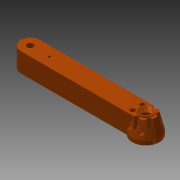
# Autodesk Inventor part: xy ubis mount arm mod
Saved by Autodesk Inventor 2013 (Build 170138000, 138)
## iProperties
Created: 2013-07-23
Part Number: xy ubis mount arm mod
Material: Generic
Document SubType Name: Modeling
Designer: employee
Density: 1 g/cm^3
Mass: 100.24 g
Surface Area: 228.044 cm^2
Volume: 100.24 cm^3
Author: employee
Autodesk Inventor part; units mm, degrees
ref_plane "YZ Plane" through (0, 0, 0) normal (1, 0, 0) x (0, 1, 0)
ref_plane "XZ Plane" through (0, 0, 0) normal (0, 1, 0) x (-1, 0, 0)
ref_plane "XY Plane" through (0, 0, 0) normal (0, 0, 1) x (1, 0, 0)
sketch "Sketch1" plane through (0, 0, 0) normal (0, 0, 1) x (1, 0, 0)
  line L0 (0, 12.5) -> (150, 12.5)
  line L1 (150, -12.5) -> (0, -12.5)
  arc A0 (0, 12.5) -> (0, -12.5) centre (0, 0) ccw
  circle A1 centre (0, 0) radius 4.05
  arc A2 (150, -12.5) -> (150, 12.5) centre (150, 0) ccw
  dimension "d0" = 12.5
  dimension "d3" = 8.1
  dimension "d121" = 150
  constraints: 4 end point, 4 point on circle, 4 tangent, 3 centre point, 2 coincident, 1 horizontal, 1 parallel
  measures "d0" radius of A0
  measures "d3" diameter of A1
  measures "d121" distance of A2.centre point (0, 0)
extrude "Extrusion1" add sketch "Sketch1" along normal blind 25
sketch "Sketch5" plane through (0, 0, 0) normal (0, 0, -1) x (-1, 0, 0)
  line L0 (0, 12.5) -> (-162.5, 12.5)
  line L1 (-162.5, 12.5) -> (-162.5, -12.5)
  line L2 (-162.5, -12.5) -> (0, -12.5)
  circle A0 centre (-150, 0) radius 12.5
  circle A1 centre (-150, 0) radius 8.1
  arc A2 (-162.5, 12.5) -> (-162.5, -12.5) centre (-150, 0) ccw projected
  dimension "d19" = 16.2
  constraints: 6 end point, 3 tangent, 2 centre point, 2 coincident, 1 other
  measures "d19" diameter of A1
extrude "Extrusion5" cut sketch "Sketch5" against normal blind 19 contours A1
sketch "Sketch17" plane through (0, 0, 0) normal (0, 0, -1) x (-1, 0, 0)
  line L0 (0, 12.5) -> (-150, 12.5) projected
  circle A0 centre (0, 0) radius 4.05 projected
  line L1 (0, 0) -> (-25, 0)
  circle A1 centre (-25, 0) radius 1.5
  point P0 (-154.6624, 12.5)
  point P1 (-154.5, 12.5)
  dimension "d85" = 25
  dimension "d86" = 3
  constraints: 2 end point, 1 centre point, 1 coincident, 1 parallel
  measures "d85" distance of L1.start L1.end
  measures "d86" diameter of A1
extrude "Extrusion16" cut sketch "Sketch17" against normal through all contours A1
sketch "Sketch26" plane through (0, 0, 25) normal (0, 0, 1) x (1, 0, 0)
  arc A0 (150, -12.5) -> (150, 12.5) centre (150, 0) ccw projected
  circle A1 centre (150, 0) radius 9
  dimension "d122" = 18
  constraints: 1 centre point, 1 coincident
  measures "d122" diameter of A1
extrude "Extrusion24" add sketch "Sketch26" along normal blind 1.5
sketch "Sketch27" plane through (0, 0, 0) normal (0, 1, 0) x (-1, 0, 0)
  line L0 (-4.05, 25) -> (-4.05, 0) projected
  line L1 (-4.05, 0) -> (-23.5, 0) projected
  line L2 (-23.5, 0) -> (-23.5, 25) projected
  line L3 (-23.5, 25) -> (-4.05, 25) projected
  line L4 (-162.5, 0) -> (-162.5, 25) projected
  line L5 (-162.5, 25) -> (-159, 25) projected
  line L6 (-159, 25) -> (-159, 26.5) projected
  line L7 (-159, 26.5) -> (-141, 26.5) projected
  line L8 (-141, 26.5) -> (-141, 25) projected
  line L9 (-141, 25) -> (-26.5, 25) projected
  line L10 (-26.5, 25) -> (-26.5, 0) projected
  line L11 (-26.5, 0) -> (-141.9, 0) projected
  line L12 (-141.9, 0) -> (-141.9, 19) projected
  line L13 (-141.9, 19) -> (-158.1, 19) projected
  line L14 (-158.1, 19) -> (-158.1, 0) projected
  line L15 (-158.1, 0) -> (-162.5, 0) projected
  line L16 (12.5, 25) -> (12.5, 0) projected
  line L17 (12.5, 0) -> (4.05, 0) projected
  line L18 (4.05, 0) -> (4.05, 25) projected
  line L19 (4.05, 25) -> (12.5, 25) projected
  line L20 (-162.5, 0) -> (-167.5, 0)
  line L21 (-167.5, 0) -> (-167.5, 5)
  line L22 (-167.5, 5) -> (-162.5, 25)
  line L23 (-150, 19) -> (-150, 26.5)
  point P0 (0, 0)
  dimension "d127" = 5
  dimension "d129" = 5
  constraints: 8 end point, 2 midpoint, 1 parallel, 1 perpendicular
  measures "d127" distance of L20.end L21.end
  measures "d129" distance of L4.start L20.end
revolve "Revolution1" add sketch "Sketch27" angle 360 about axis through (150, 0, 19) along (0, 0, 1) contours L20 L21 L22 L4
sketch "Sketch28" plane through (0, 0, 25) normal (0, 0, 1) x (1, 0, 0)
  circle A0 centre (150, 0) radius 9 projected
  line L0 (0, -12.5) -> (150, -12.5) projected
  circle A1 centre (139.1747, 6.25) radius 3
  line L1 (139.1747, 6.25) -> (150, 0)
  dimension "d131" = 30
  dimension "d132" = 12.5
  dimension "d134" = 6
  constraints: 2 end point, 1 centre point, 1 coincident
  measures "d131" angle of L0 L1
  measures "d132" distance of L1.start L1.end
  measures "d134" diameter of A1
extrude "Extrusion25" cut sketch "Sketch28" against normal blind 20 contours A1
sketch "Sketch29" plane through (139.1747, 6.25, 5) normal (0, 0, 1) x (1, 0, 0)
  circle A0 centre (0, 0) radius 3 projected
  circle A1 centre (0, 0) radius 1.6
  point P0 (-139.1747, -6.25)
  dimension "d137" = 3.2
  constraints: 1 centre point, 1 coincident
  measures "d137" diameter of A1
extrude "Extrusion26" cut sketch "Sketch29" against normal through all contours A1
pattern_circular "Circular Pattern1" count 6 over 360 about axis through (150, 0, 15) along (0, 0, 1) of "Extrusion26", "Extrusion25"
sketch "Sketch30" plane through (0, 12.5, 25) normal (0, 1, 0) x (1, 0, 0)
  line L0 (0, 25) -> (0, 0) projected
  line L1 (141, -1.5) -> (159, -1.5) projected
  line L2 (142.75, 12.5) -> (157.25, 12.5)
  circle A0 centre (142.75, 12.5) radius 3
  circle A1 centre (157.25, 12.5) radius 3
  point P0 (150, -1.5)
  point P1 (150, 12.5)
  point P2 (0, 12.5)
  dimension "d144" = 14.5
  dimension "d146" = 6
  constraints: 3 midpoint, 2 centre point, 2 coincident, 2 end point, 1 equal radius, 1 horizontal alignment, 1 parallel, 1 vertical alignment
  measures "d144" distance of L2.start L2.end
  measures "d146" diameter of A1
extrude "Extrusion27" cut sketch "Sketch30" along normal through all
sketch "Sketch31" plane through (0, 12.5, 25) normal (0, 1, 0) x (1, 0, 0)
  arc A0 (159.9281, 13.852) -> (158.1229, 9.6298) centre (157.25, 12.5) ccw projected
  arc A1 (141.8771, 9.6298) -> (140.0719, 13.852) centre (142.75, 12.5) ccw projected
  circle A2 centre (142.75, 12.5) radius 1.6
  circle A3 centre (157.25, 12.5) radius 1.6
  point P0 (0, 25)
  dimension "d149" = 3.2
  constraints: 2 centre point, 2 coincident, 1 equal radius
  measures "d149" diameter of A3
extrude "Extrusion28" cut sketch "Sketch31" against normal through all
sketch "Sketch32" plane through (0, -12.5, 0) normal (0, -1, 0) x (1, 0, 0)
  circle A0 centre (142.75, 12.5) radius 1.6 projected
  circle A1 centre (157.25, 12.5) radius 1.6 projected
  line L0 (148.4, 5) -> (148.4, 0) projected
  line L1 (148.4, 0) -> (137.7526, 0) projected
  line L2 (137.7526, 0) -> (137.7526, 5) projected
  line L3 (147, 25) -> (147, 23.5802) projected
  line L4 (0, 25) -> (147, 25) projected
  line L5 (0, 0) -> (0, 25) projected
  line L6 (137.7526, 0) -> (0, 0) projected
  line L7 (147, 5) -> (148.4, 5) projected
  line L8 (147, 23.5802) -> (147, 5) projected
  line L9 (151.6, 0) -> (151.6, 5) projected
  line L10 (151.6, 5) -> (153, 5) projected
  line L11 (153, 5) -> (153, 23.5802) projected
  line L12 (162.2474, 5) -> (162.2474, 0) projected
  line L13 (162.2474, 0) -> (151.6, 0) projected
  line L14 (145.9832, 12.5) -> (144.3666, 9.7)
  line L15 (144.3666, 9.7) -> (141.1334, 9.7)
  line L16 (141.1334, 9.7) -> (139.5168, 12.5)
  line L17 (139.5168, 12.5) -> (141.1334, 15.3)
  line L18 (141.1334, 15.3) -> (144.3666, 15.3)
  line L19 (144.3666, 15.3) -> (145.9832, 12.5)
  line L20 (160.4832, 12.5) -> (158.8666, 9.7)
  line L21 (158.8666, 9.7) -> (155.6334, 9.7)
  line L22 (155.6334, 9.7) -> (154.0168, 12.5)
  line L23 (154.0168, 12.5) -> (155.6334, 15.3)
  line L24 (155.6334, 15.3) -> (158.8666, 15.3)
  line L25 (158.8666, 15.3) -> (160.4832, 12.5)
  dimension "d153" = 5.6
  constraints: 24 end point, 2 coincident, 2 horizontal, 1 collinear, 28 other
  measures "d153" distance between parallel lines of L21 L24
extrude "Extrusion29" cut sketch "Sketch32" against normal blind 2.5 and the other way blind 25 contours L14 L15 L16 L17 L18 L19 | L20 L21 L22 L23 L24 L25
sketch "Sketch33" plane through (0, 12.5, 25) normal (0, 1, 0) x (1, 0, 0)
  circle A0 centre (142.75, 12.5) radius 1.6 projected
  arc A1 (141.8771, 9.6298) -> (140.0719, 13.852) centre (142.75, 12.5) ccw projected
  circle A2 centre (142.75, 12.5) radius 3
  circle A3 centre (157.25, 12.5) radius 1.6 projected
  arc A4 (159.9281, 13.852) -> (158.1229, 9.6298) centre (157.25, 12.5) ccw projected
  circle A5 centre (157.25, 12.5) radius 3
  constraints: 2 coincident, 7 other
extrude "Extrusion30" cut sketch "Sketch33" against normal blind 2.5
sketch "Sketch34" plane through (150, 0, 26.5) normal (0, 0, 1) x (1, 0, 0)
  circle A0 centre (0, 0) radius 9 projected
  circle A1 centre (0, 0) radius 6.95
  point P0 (-150, 0)
  dimension "d160" = 13.9
  constraints: 1 centre point, 1 coincident
  measures "d160" diameter of A1
extrude "Extrusion31" cut sketch "Sketch34" against normal through all contours A1
sketch "Sketch35" plane through (150, 0, 19) normal (0, 0, -1) x (-1, 0, 0)
  circle A0 centre (0, 0) radius 8.1 projected
  point P0 (150, 0)
extrude "Extrusion32" cut sketch "Sketch35" against normal through all draft -45
sketch "Sketch36" plane through (0, 0, 0) normal (0, 1, 0) x (-1, 0, 0)
  line L0 (12.5, 0) -> (4.05, 0) projected
  line L1 (4.05, 0) -> (4.05, 25) projected
  line L2 (4.05, 25) -> (12.5, 25) projected
  line L3 (12.5, 25) -> (12.5, 0) projected
  line L4 (-4.05, 0) -> (-23.5, 0) projected
  line L5 (-23.5, 0) -> (-23.5, 25) projected
  line L6 (-23.5, 25) -> (-4.05, 25) projected
  line L7 (-4.05, 25) -> (-4.05, 0) projected
  line L8 (-141, 26.5) -> (-141, 25) projected
  line L9 (-141, 25) -> (-26.5, 25) projected
  line L10 (-26.5, 25) -> (-26.5, 0) projected
  line L11 (-26.5, 0) -> (-141.9, 0) projected
  line L12 (-141.9, 0) -> (-141.9, 11.1445) projected
  arc A0 (-141.9, 11.1445) -> (-141.9, 13.8555) centre (-142.75, 12.5) ccw projected
  line L13 (-141.9, 13.8555) -> (-141.9, 19) projected
  line L14 (-141.9, 19) -> (-143.05, 20.15) projected
  line L15 (-143.05, 20.15) -> (-143.05, 26.5) projected
  line L16 (-143.05, 26.5) -> (-141, 26.5) projected
  line L17 (-159, 25) -> (-159, 26.5) projected
  line L18 (-159, 26.5) -> (-156.95, 26.5) projected
  line L19 (-156.95, 26.5) -> (-156.95, 20.15) projected
  line L20 (-156.95, 20.15) -> (-158.1, 19) projected
  line L21 (-158.1, 19) -> (-158.1, 13.8555) projected
  arc A1 (-158.1, 13.8555) -> (-158.1, 11.1445) centre (-157.25, 12.5) ccw projected
  line L22 (-158.1, 11.1445) -> (-158.1, 0) projected
  line L23 (-158.1, 0) -> (-167.5, 0) projected
  line L24 (-167.5, 0) -> (-167.5, 5) projected
  line L25 (-167.5, 5) -> (-162.5, 25) projected
  line L26 (-162.5, 25) -> (-159, 25) projected
  line L27 (-156.95, 26.5) -> (-156.95, 28.5)
  line L28 (-156.95, 28.5) -> (-157.95, 27.5)
  line L29 (-157.95, 27.5) -> (-156.95, 26.5)
  line L30 (-156.95, 26.5) -> (-143.05, 26.5)
  line L31 (-150, 26.5) -> (-150, 31.1072)
  point P0 (0, 0)
  dimension "d166" = 2
  constraints: 10 end point, 4 perpendicular, 1 midpoint, 1 parallel
  measures "d166" distance of L18.end L27.end
coil "Coil3" sketch "Sketch36" operation cut axis through (150, 0, 26.5) along (0, 0, -1) pitch 2.0001 turns 10 hand right contours L29 L28 L27
body "Solid1"
